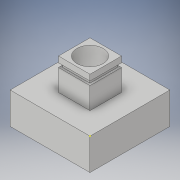
# Autodesk Inventor part: Hydraulic cylinder part 1
Saved by Autodesk Inventor 2018 (Build 220112000, 112)
## iProperties
Created: 2018-07-18
Part Number: Hydraulic cylinder part 1
Material: Generic
Document SubType Name: Modeling
Designer: BB-8
Density: 1 g/cm^3
Appearance: Default
Author: BB-8
Autodesk Inventor part; units mm, degrees
ref_plane "YZ Plane" through (0, 0, 0) normal (1, 0, 0) x (0, 1, 0)
ref_plane "XZ Plane" through (0, 0, 0) normal (0, 1, 0) x (-1, 0, 0)
ref_plane "XY Plane" through (0, 0, 0) normal (0, 0, 1) x (1, 0, 0)
sketch "Sketch1" plane through (0, 0, 0) normal (0, 1, 0) x (-1, 0, 0)
  line L0 (0, 0) -> (76, 0)
  line L1 (76, 0) -> (76, -76)
  line L2 (76, -76) -> (0, -76)
  line L3 (0, -76) -> (0, 0)
  dimension "d0" = 76
  dimension "d1" = 76
  constraints: 8 end point, 2 parallel, 1 horizontal, 1 perpendicular
  measures "d0" distance of L1.end L2.end
  measures "d1" distance of L0.end L1.end
extrude "Extrusion1" add sketch "Sketch1" along normal blind 30
sketch "Sketch2" plane through (0, 30, 0) normal (0, 1, 0) x (1, 0, 0)
  point P0 (0, 0)
sketch "Sketch3" plane through (0, 30, 0) normal (0, 1, 0) x (1, 0, 0)
  line L0 (-51, 21) -> (-21, 21)
  line L1 (-21, 21) -> (-21, 51)
  line L2 (-21, 51) -> (-51, 51)
  line L3 (-51, 51) -> (-51, 21)
  point P0 (0, 0)
  dimension "d4" = 30
  dimension "d5" = 30
  constraints: 8 end point, 2 parallel, 1 horizontal, 1 perpendicular
  measures "d4" distance of L2.end L1.end
  measures "d5" distance of L1.end L0.end
extrude "Extrusion2" add sketch "Sketch3" along normal blind 30
sketch "Sketch4" plane through (-21, 30, -21) normal (1, 0, 0) x (0, 0, -1)
  line L0 (30, 0) -> (30, 30) projected
  line L1 (0, 20.6) -> (30, 20.6)
  line L2 (30, 20.6) -> (30, 24.4)
  line L3 (30, 24.4) -> (0, 24.4)
  line L4 (0, 24.4) -> (0, 20.6)
  point P0 (-21, -30)
  point P1 (0, 22.5)
  point P2 (30, 22.5)
  dimension "d8" = 3.8
  constraints: 8 end point, 2 parallel, 2 point on line, 1 horizontal, 1 perpendicular
  measures "d8" distance of L2.end L1.end
sketch "Sketch5" plane through (-21, 30, -51) normal (0, 0, -1) x (-1, 0, 0)
  line L0 (30, 0) -> (30, 30) projected
  line L1 (0, 20.6) -> (30, 20.6)
  line L2 (30, 20.6) -> (30, 24.4)
  line L3 (30, 24.4) -> (0, 24.4)
  line L4 (0, 24.4) -> (0, 20.6)
  line L5 (0, 20.6) -> (30, 24.4) construction
  line L6 (30, 20.6) -> (0, 24.4) construction
  point P0 (-21, -30)
  point P1 (30, 22.5)
  point P2 (15, 22.5)
  dimension "d9" = 3.8
  constraints: 12 end point, 2 midpoint, 2 parallel, 2 point on line, 1 horizontal, 1 perpendicular
  measures "d9" distance of L2.end L1.end
sketch "Sketch6" plane through (-51, 30, -51) normal (-1, 0, 0) x (0, 0, 1)
  line L0 (30, 0) -> (30, 30) projected
  line L1 (0, 20.6) -> (30, 20.6)
  line L2 (30, 20.6) -> (30, 24.4)
  line L3 (30, 24.4) -> (0, 24.4)
  line L4 (0, 24.4) -> (0, 20.6)
  line L5 (0, 20.6) -> (30, 24.4) construction
  line L6 (30, 20.6) -> (0, 24.4) construction
  point P0 (51, -30)
  point P1 (15, 22.5)
  dimension "d10" = 3.8
  constraints: 12 end point, 2 midpoint, 2 parallel, 1 horizontal, 1 perpendicular, 1 point on line
  measures "d10" distance of L2.end L1.end
sketch "Sketch7" plane through (-51, 30, -21) normal (0, 0, 1) x (1, 0, 0)
  line L0 (30, 0) -> (30, 30) projected
  line L1 (0, 24.4) -> (30, 24.4)
  line L2 (30, 24.4) -> (30, 20.6)
  line L3 (30, 20.6) -> (0, 20.6)
  line L4 (0, 20.6) -> (0, 24.4)
  line L5 (0, 24.4) -> (30, 20.6) construction
  line L6 (30, 24.4) -> (0, 20.6) construction
  point P0 (51, -30)
  point P1 (15, 22.5)
  dimension "d11" = 3.8
  constraints: 12 end point, 2 midpoint, 2 parallel, 1 horizontal, 1 perpendicular, 1 point on line
  measures "d11" distance of L1.end L2.end
extrude "Extrusion3" cut sketch "Sketch6" against normal blind 2
extrude "Extrusion4" cut sketch "Sketch7" against normal blind 2
extrude "Extrusion5" cut sketch "Sketch4" against normal blind 2
extrude "Extrusion6" cut sketch "Sketch5" against normal blind 2
sketch "Sketch8" plane through (0, 60, 0) normal (0, 1, 0) x (1, 0, 0)
  line L0 (-21, 21) -> (-51, 21) projected
  line L1 (-21, 51) -> (-21, 21) projected
  circle A0 centre (-36, 36) radius 12.5
  point P0 (0, 0)
  dimension "d20" = 25
  constraints: 1 centre point
  measures "d20" diameter of A0
extrude "Extrusion7" cut sketch "Sketch8" against normal blind 25
body "Solid1"
